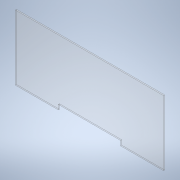
# Autodesk Inventor part: Acrilico1_Prensa
Saved by Autodesk Inventor 2021 (Build 250183000, 183)
## iProperties
Created: 2021-08-02
Part Number: Acrilico1_Prensa
Material: PMMA Plastic
Document SubType Name: Modeling
Designer: Nelson
Density: 1.188 g/cm^3
Appearance: Polycarbonate - Clear
Author: Nelson
Autodesk Inventor part; units mm, degrees
ref_plane "YZ Plane" through (0, 0, 0) normal (1, 0, 0) x (0, 1, 0)
ref_plane "XZ Plane" through (0, 0, 0) normal (0, 1, 0) x (-1, 0, 0)
ref_plane "XY Plane" through (0, 0, 0) normal (0, 0, 1) x (1, 0, 0)
sketch "Sketch1" plane through (0, 0, 0) normal (0, 0, 1) x (1, 0, 0)
  line L0 (1250.8, 0) -> (1250.8, 549.6)
  line L1 (1250.8, 549.6) -> (0, 549.6)
  line L2 (0, 549.6) -> (0, 0)
  line L3 (0, 0) -> (362, 0)
  line L4 (362, 0) -> (362, 40)
  line L5 (1250.8, 0) -> (888.8, 0)
  line L6 (888.8, 0) -> (888.8, 40)
  line L7 (362, 40) -> (888.8, 40)
  dimension "d0" = 1250.8
  dimension "d1" = 549.6
  dimension "d4" = 362
  dimension "d5" = 40
  dimension "d6" = 362
  dimension "d7" = 40
  dimension "d8" = 549.6
  constraints: 16 end point, 3 horizontal, 2 perpendicular, 1 parallel
  measures "d0" distance of L1.end L0.end
  measures "d1" distance of L0.start L0.end
  measures "d4" distance of L2.end L3.end
  measures "d5" distance of L3.end L4.end
  measures "d6" distance of L0.start L5.end
  measures "d7" distance of L5.end L6.end
  measures "d8" distance of L1.end L2.end
extrude "Extrusion1" add sketch "Sketch1" against normal blind 10
equation "\"d6\" = d4"
equation "\"d7\" = d5"
equation "\"d8\" = d1"
body "Solid1"
